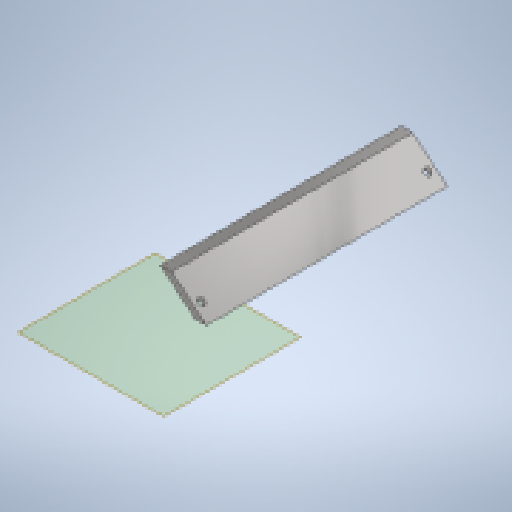
# Autodesk Inventor part: strug
Saved by Autodesk Inventor 2023.5 (Build 275446000, 446)
## iProperties
Created: 2022-12-26
Part Number: strug
Material: Steel, Alloy
Document SubType Name: Modeling
Designer: Kamil
Density: 7.73 g/cm^3
Appearance: Semi-Polished
Author: Kamil
Autodesk Inventor part; units mm, degrees
ref_plane "YZ Plane" through (0, 0, 0) normal (1, 0, 0) x (0, 1, 0)
ref_plane "XZ Plane" through (0, 0, 0) normal (0, 1, 0) x (-1, 0, 0)
ref_plane "XY Plane" through (0, 0, 0) normal (0, 0, 1) x (1, 0, 0)
sketch "Sketch1" plane through (0, 0, 0) normal (0, 0, 1) x (1, 0, 0)
  line L0 (10.7451, 5.5) -> (50.1922, -27.6) projected
  line L1 (50.1922, -27.6) -> (100, -27.6) projected
  line L2 (100, -27.6) -> (100, -23.6) projected
  line L3 (100, -23.6) -> (83.9, -23.6) projected
  arc A0 (65.8, -5.5) -> (83.9, -23.6) centre (83.9, -5.5) ccw projected
  line L4 (65.8, -5.5) -> (65.8, 5.5) projected
  line L5 (65.8, 5.5) -> (10.7451, 5.5) projected
  line L6 (7.1699, 8.5) -> (10.7451, 5.5) projected
  line L7 (65.8, 5.5) -> (10.7451, 5.5) projected
  line L8 (65.8, 5.5) -> (65.8, 8.5) projected
  line L9 (65.8, 8.5) -> (7.1699, 8.5) projected
  circle A1 centre (83.9, -5.5) radius 16.1 projected
  line L10 (83.9, 10.6) -> (-17.1951, 10.6)
  line L11 (100, -5.5) -> (0, -5.5)
  line L12 (0, -5.5) -> (0, 10.6)
  line L13 (7.1699, 8.5) -> (4.6672, 10.6)
  line L14 (7.1699, 8.5) -> (5.2415, 6.2019)
  line L15 (5.2415, 6.2019) -> (0, 10.6)
  line L16 (0, 10.6) -> (22.9813, -8.6836)
  line L17 (22.9813, -8.6836) -> (24.9097, -6.3855)
  point P0 (0, 0)
  dimension "d0" = 100
  dimension "d1" = 3
  dimension "d2" = 30
  constraints: 16 end point, 4 point on line, 3 perpendicular, 2 horizontal, 2 point on circle, 1 collinear
  measures "d0" distance of L11.start L11.end
  measures "d1" distance of L6.start L14.end
  measures "d2" distance of L12.end L16.end
extrude "Extrusion1" add sketch "Sketch1" against normal blind 100 contours L17 L16 L11 L0 | L11 L16 L14 L6 L0 | L14 L15 L10 L13
ref_plane "Work Plane1" through (8.1777, -6.0133, 8.6215) normal (0, -1, 0) x (0, 0, 1)
sketch "Sketch2" plane through (8.1777, -6.0133, 8.6215) normal (0, -1, 0) x (0, 0, 1)
  line L0 (-22.0032, -27.7487) -> (35.8312, 20.7819)
  line L1 (35.8312, 20.7819) -> (3.0626, 38.2053)
  line L2 (3.0626, 38.2053) -> (-26.1922, -24.5344)
  line L3 (-26.1922, -24.5344) -> (-22.0032, -27.7487)
  line L4 (-46.8404, -23.7111) -> (-15.3118, 43.9022)
  line L5 (-15.3118, 43.9022) -> (-51.9953, 38.492)
  line L6 (-51.9953, 38.492) -> (-51.9953, -22.5683)
  line L7 (-51.9953, -22.5683) -> (-46.8404, -23.7111)
  line L8 (-70.2281, -23.6979) -> (-65.0733, -22.5551)
  line L9 (-65.0733, -22.5551) -> (-65.0733, 38.4893)
  line L10 (-94.9551, 29.3293) -> (-70.2281, -23.6979)
  line L11 (-65.0733, 38.4893) -> (-94.9551, 29.3293)
  line L12 (-90.9709, -24.4596) -> (-115.5317, 28.2112)
  arc A0 (-115.5317, 28.2112) -> (-139.4308, 9.4739) centre (-87.2125, -32.5195) ccw
  line L13 (-139.4308, 9.4739) -> (-95.1598, -27.6739)
  line L14 (-95.1598, -27.6739) -> (-90.9709, -24.4596)
  point P0 (-8.6215, 8.1777)
  point P1 (-24.0977, -26.1415)
  point P2 (-49.4178, -23.1397)
  point P3 (-67.6507, -23.1265)
  point P4 (-93.0654, -26.0667)
  constraints: 30 end point, 2 point on circle, 1 centre point
ref_plane "Work Plane2" through (40.3431, -2.6133, -6) normal (0, -1, 0) x (1, 0, 0)
extrude "Extrusion2" cut sketch "Sketch2" against normal up to surface (3.4 mm away)
extrude "Extrusion3" cut sketch "Sketch2" along normal blind 1
sketch "Sketch3" plane through (15.747, -2.6133, 0) normal (0, -1, 0) x (1, 0, 0)
  line L0 (4.6672, 0) -> (4.6672, -11.8362) projected
  line L1 (0, 0) -> (4.6672, 0) projected
  line L2 (0, -9.66) -> (0, 0) projected
  line L3 (4.6672, -11.8362) -> (0, -9.66) projected
  line L4 (4.6672, -32.8682) -> (4.6672, -43.3737) projected
  line L5 (0, -30.6918) -> (4.6672, -32.8682) projected
  line L6 (0, -43.3737) -> (0, -30.6918) projected
  line L7 (4.6672, -43.3737) -> (0, -43.3737) projected
  line L8 (4.6672, -56.4518) -> (4.6672, -66.9512) projected
  line L9 (0, -56.4518) -> (4.6672, -56.4518) projected
  line L10 (0, -69.1275) -> (0, -56.4518) projected
  line L11 (4.6672, -66.9512) -> (0, -69.1275) projected
  line L12 (4.6672, -88.0491) -> (4.6672, -100) projected
  line L13 (0, -90.2254) -> (4.6672, -88.0491) projected
  line L14 (0, -100) -> (0, -90.2254) projected
  line L15 (4.6672, -100) -> (0, -100) projected
  line L16 (0, -90.2254) -> (12.0968, -84.5846)
  line L17 (0, -90.2254) -> (4.6672, -88.0491) projected
  line L18 (12.0968, -84.5846) -> (12.0968, -100)
  line L19 (4.6672, -100) -> (0, -100) projected
  line L20 (12.0968, -100) -> (0, -100)
  line L21 (8.636, -100) -> (8.636, -86.1984) projected
  line L22 (8.636, -86.1984) -> (9.1627, -85.9528) projected
  line L23 (9.1627, -64.8548) -> (9.1627, -85.9528) projected
  line L24 (9.1627, -64.8548) -> (8.636, -65.1005) projected
  line L25 (8.636, -65.1005) -> (8.636, -56.4518) projected
  line L26 (8.636, -56.4518) -> (9.1627, -56.4518) projected
  line L27 (9.1627, -43.3737) -> (9.1627, -56.4518) projected
  line L28 (9.1627, -43.3737) -> (8.636, -43.3737) projected
  line L29 (8.636, -43.3737) -> (8.636, -34.7188) projected
  line L30 (8.636, -34.7188) -> (9.1627, -34.9645) projected
  line L31 (9.1627, -13.9325) -> (9.1627, -34.9645) projected
  line L32 (9.1627, -13.9325) -> (8.636, -13.6868) projected
  line L33 (8.636, -13.6868) -> (8.636, 0) projected
  line L34 (7.2344, 0) -> (8.636, 0) projected
  line L35 (7.2344, 0) -> (7.2344, -100) projected
  line L36 (8.636, -100) -> (7.2344, -100) projected
  line L37 (0, -30.6918) -> (5.2437, -33.137) projected
  line L38 (5.2437, -33.137) -> (5.2437, -43.3737) projected
  line L39 (5.2437, -43.3737) -> (0, -43.3737) projected
  line L40 (0, -43.3737) -> (0, -30.6918) projected
  line L41 (5.2437, -66.6823) -> (0, -69.1275) projected
  line L42 (0, -69.1275) -> (0, -56.4518) projected
  line L43 (0, -56.4518) -> (5.2437, -56.4518) projected
  line L44 (5.2437, -56.4518) -> (5.2437, -66.6823) projected
  line L45 (5.2437, -87.7803) -> (5.2437, -100) projected
  line L46 (7.2344, -100) -> (5.2437, -100) projected
  line L47 (7.2344, 0) -> (7.2344, -100) projected
  line L48 (5.2437, 0) -> (7.2344, 0) projected
  line L49 (5.2437, 0) -> (5.2437, -12.1051) projected
  line L50 (5.2437, -12.1051) -> (0, -9.66) projected
  line L51 (0, -9.66) -> (0, 0) projected
  line L52 (-15.747, 0) -> (0, 0) projected
  line L53 (-15.747, 0) -> (-15.747, -100) projected
  line L54 (0, -100) -> (-15.747, -100) projected
  line L55 (0, -100) -> (0, -90.2254) projected
  line L56 (0, -90.2254) -> (5.2437, -87.7803) projected
  line L57 (4.6672, -66.9512) -> (0, -69.1275) projected
  line L58 (0, -69.1275) -> (9.1627, -64.8548)
  line L59 (9.1627, -56.4518) -> (4.6672, -56.4518) projected
  line L60 (9.1627, -56.4518) -> (9.1627, -64.8548)
  line L61 (0, -56.4518) -> (9.1627, -56.4518)
  line L62 (0, -43.3737) -> (9.1627, -43.3737)
  line L63 (8.636, -34.7188) -> (9.1627, -34.9645) projected
  line L64 (9.1627, -34.9645) -> (9.1627, -43.3737)
  line L65 (8.636, -43.3737) -> (8.636, -34.7188) projected
  line L66 (0, -30.6918) -> (4.6672, -32.8682) projected
  line L67 (0, -30.6918) -> (9.1627, -34.9645)
  line L68 (4.6672, -11.8362) -> (0, -9.66) projected
  line L69 (4.6672, -11.8362) -> (9.1627, -13.9325)
  line L70 (9.1627, -13.9325) -> (9.1627, 0)
  line L71 (9.1627, 0) -> (0, 0)
  line L72 (4.6672, 0) -> (-11.0798, 0) projected
  line L73 (8.9504, 0) -> (9.1627, -0.253) projected
  line L74 (9.1627, 0) -> (9.1627, -0.253) projected
  line L75 (8.9504, 0) -> (9.1627, 0) projected
  line L76 (9.1627, -99.5783) -> (8.8088, -100) projected
  line L77 (9.1627, -100) -> (8.8088, -100) projected
  line L78 (9.1627, -99.5783) -> (9.1627, -100) projected
  point P0 (-15.747, 0)
  point P1 (8.9504, 0)
  point P2 (5.2437, -12.1051)
  point P3 (7.2344, 0)
  point P4 (5.2437, -33.137)
  point P5 (5.2437, -43.3737)
  point P6 (5.2437, -66.6823)
  point P7 (5.2437, -87.7803)
  point P8 (5.2437, -100)
  point P9 (8.636, -100)
  point P10 (8.636, -86.1984)
  constraints: 24 end point, 5 collinear, 3 perpendicular, 2 parallel, 1 point on line, 1 vertical
extrude "Extrusion4" cut sketch "Sketch3" along normal through all contours L48 L35 L69 L49 | L34 L33 L69 L35 | L67 L29 L62 L35 | L35 L62 L38 L67 | L71 L70 L73 | L59 L25 L58 L35 | L35 L58 L44 L59 | L45 L16 L35 L20 | L16 L21 L20 L35 | L76 L78 L20
sketch "Sketch4" plane through (0, 10.6, -100) normal (-0.6427876, -0.7660444, 0) x (0.7660444, -0.6427876, 0)
  line L0 (30, 34.2459) -> (20.5562, 30.8725) projected
  line L1 (20.5562, 30.8725) -> (20.5562, 43.5482) projected
  line L2 (20.5562, 43.5482) -> (30, 43.5482) projected
  line L3 (30, 56.6263) -> (30, 43.5482) projected
  line L4 (30, 56.6263) -> (20.5562, 56.6263) projected
  line L5 (20.5562, 56.6263) -> (20.5562, 69.3082) projected
  line L6 (20.5562, 69.3082) -> (30, 65.9347) projected
  line L7 (30, 86.9667) -> (30, 65.9347) projected
  line L8 (30, 86.9667) -> (20.5562, 90.34) projected
  line L9 (20.5562, 90.34) -> (20.5562, 100) projected
  line L10 (0, 100) -> (20.5562, 100) projected
  line L11 (0, 100) -> (0, 0) projected
  line L12 (20.5562, 0) -> (0, 0) projected
  line L13 (20.5562, 0) -> (20.5562, 9.7746) projected
  line L14 (20.5562, 9.7746) -> (30, 13.148) projected
  line L15 (30, 34.2459) -> (30, 13.148) projected
  line L16 (73.894, 94) -> (30.9766, 94)
  line L17 (24.1315, 94) -> (11.5095, 94)
  line L18 (31.2695, 94) -> (24.1315, 94)
  line L19 (0, 100) -> (0, 0) projected
  line L20 (0, 50) -> (30, 50.0873)
  line L21 (20.5562, 100) -> (18.5562, 100)
  line L22 (18.5562, 100) -> (18.5562, 94)
  line L23 (18.5562, 94) -> (20.5562, 94)
  line L24 (20.5562, 94) -> (20.5562, 100)
  circle A0 centre (15.5562, 97) radius 3
  circle A1 centre (15.5562, 97) radius 1.5
  circle A2 centre (15.8294, 3.0913) radius 1.5
  point P0 (6.8135, 100)
  dimension "d11" = 2
  dimension "d12" = 3
  constraints: 16 end point, 4 horizontal, 3 centre point, 3 tangent, 2 midpoint, 2 parallel, 1 coincident, 1 perpendicular, 1 point on line, 1 symmetric about line, 6 other
  measures "d11" distance of L23.end L22.end
  measures "d12" diameter of A1
extrude "Extrusion5" cut sketch "Sketch4" against normal blind 10 contours A1 | A2
chamfer "Chamfer1" distance 1 angle 45 2 edges at (10.9769, 1.3893, -96.9087) (10.7677, 1.5648, -3)
sketch "Szkic5" plane through (15.747, -2.6133, 0) normal (0, -1, 0) x (1, 0, 0)
  line L0 (4.6672, 0) -> (4.6672, -11.8362) projected
  line L1 (0, 0) -> (4.6672, 0) projected
  line L2 (0, -9.66) -> (0, 0) projected
  line L3 (4.6672, -11.8362) -> (0, -9.66) projected
  line L4 (4.6672, -32.8682) -> (4.6672, -43.3737) projected
  line L5 (0, -30.6918) -> (4.6672, -32.8682) projected
  line L6 (0, -43.3737) -> (0, -30.6918) projected
  line L7 (4.6672, -43.3737) -> (0, -43.3737) projected
  line L8 (4.6672, -56.4518) -> (4.6672, -66.9512) projected
  line L9 (0, -56.4518) -> (4.6672, -56.4518) projected
  line L10 (0, -69.1275) -> (0, -56.4518) projected
  line L11 (4.6672, -66.9512) -> (0, -69.1275) projected
  line L12 (4.6672, -88.0491) -> (4.6672, -100) projected
  line L13 (0, -90.2254) -> (4.6672, -88.0491) projected
  line L14 (0, -100) -> (0, -90.2254) projected
  line L15 (4.6672, -100) -> (0, -100) projected
  line L16 (4.6672, 0) -> (4.6672, -11.8362) projected
  line L17 (4.6672, 0) -> (-31.1129, 0)
  line L18 (-31.1129, 0) -> (-31.1129, -100)
  line L19 (-31.1129, -100) -> (4.6672, -100)
  line L20 (4.6672, -100) -> (4.6672, 0)
  line L21 (4.6672, -100) -> (0, -100) projected
  line L22 (4.6672, 0) -> (-11.0798, 0) projected
  line L23 (4.6672, 0) -> (18.0688, 0)
  line L24 (18.0688, 0) -> (18.0688, -100)
  line L25 (18.0688, -100) -> (4.6672, -100)
  line L26 (4.6672, -100) -> (4.6672, 0)
  point P0 (-15.747, 0)
  point P1 (4.6672, -100)
  constraints: 16 end point, 4 parallel, 2 collinear, 2 horizontal, 2 perpendicular
extrude "Wyciągnięcie proste6" cut sketch "Szkic5" along normal blind 10
ref_plane "Płaszczyzna konstrukcyjna3" through (19.0877, -1.5003, -6) normal (0, -1, 0) x (1, 0, 0)
extrude "Wyciągnięcie proste7" cut sketch "Szkic5" against normal up to surface (1.113 mm away)
sketch "Szkic6" plane through (0, 0, 0) normal (0, 0, 1) x (1, 0, 0)
  line L0 (14.4205, -1.5003) -> (19.0877, -1.5003) projected
  line L1 (19.0877, -1.5003) -> (4.6672, 10.6) projected
  line L2 (4.6672, 10.6) -> (0, 10.6) projected
  line L3 (0, 10.6) -> (14.4205, -1.5003) projected
  line L4 (0, 10.6) -> (15.3209, -2.2558)
  line L5 (15.3209, -2.2558) -> (17.2493, 0.0424)
  line L6 (19.0877, -1.5003) -> (4.6672, 10.6) projected
  point P0 (0, 0)
  point P1 (15.9548, -1.5003)
  dimension "d22" = 20
  constraints: 4 end point, 1 collinear, 1 perpendicular, 1 point on line
  measures "d22" distance of L2.end L4.end
extrude "Wyciągnięcie proste8" cut sketch "Szkic6" against normal through all contours L5 L1 L0
extrude "Wyciągnięcie proste9" add sketch "Szkic6" against normal up to surface (100 mm away) contours L0 L5 L4
body "Solid1"
